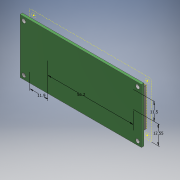
# Autodesk Inventor part: LCD Display
Saved by Autodesk Inventor 2017 (Build 210142000, 142)
## iProperties
Created: 2017-07-31
Part Number: LCD Display
Material: Generic
Document SubType Name: Modeling
Designer: AlexS
Density: 1 g/cm^3
Appearance: Default
Author: AlexS
Autodesk Inventor part; units mm, degrees
ref_plane "YZ Plane" through (0, 0, 0) normal (1, 0, 0) x (0, 1, 0)
ref_plane "XZ Plane" through (0, 0, 0) normal (0, 1, 0) x (-1, 0, 0)
ref_plane "XY Plane" through (0, 0, 0) normal (0, 0, 1) x (1, 0, 0)
sketch "Sketch1" plane through (0, 0, 0) normal (0, 1, 0) x (-1, 0, 0)
  line L0 (-40, 18) -> (40, 18)
  line L1 (40, 18) -> (40, -18)
  line L2 (40, -18) -> (-40, -18)
  line L3 (-40, -18) -> (-40, 18)
  line L4 (-40, 18) -> (40, -18) construction
  line L5 (40, 18) -> (-40, -18) construction
  point P0 (0, 0)
  dimension "d0" = 80
  dimension "d1" = 36
  constraints: 12 end point, 2 midpoint, 2 parallel, 1 horizontal, 1 perpendicular
  measures "d0" distance of L1.end L2.end
  measures "d1" distance of L0.end L1.end
extrude "Extrusion1" add sketch "Sketch1" along normal blind 1.6
sketch "Sketch2" plane through (0, 1.6, 0) normal (0, 1, 0) x (1, 0, 0)
  line L0 (-40, -18) -> (40, -18) construction
  line L1 (40, -18) -> (40, 18) construction
  line L2 (40, 18) -> (-40, 18) construction
  line L3 (-40, 18) -> (-40, -18) construction
  point P0 (0, 0)
  point P1 (-37.5, 15.5)
  point P2 (37.5, 15.5)
  point P3 (-37.5, -15.5)
  point P4 (37.5, -15.5)
  dimension "d4" = 75
  dimension "d5" = 31
  dimension "d6" = 2.5
  dimension "d7" = 2.5
  constraints: 2 horizontal alignment, 2 vertical alignment
  measures "d4" distance of point (37.5, 15.5) point (-37.5, 15.5)
  measures "d5" distance of point (-37.5, 15.5) point (-37.5, -15.5)
  measures "d6" distance from line of L3 point (-37.5, 15.5)
  measures "d7" distance from line of L2 point (-37.5, 15.5)
hole "Hole1" at (-37.5, 1.6, -15.5) at (37.5, 1.6, -15.5) at (-37.5, 1.6, 15.5) at (37.5, 1.6, 15.5) direction (0, -1, 0) diameter 2.5 end through all
sketch "Sketch3" plane through (0, 1.6, 0) normal (0, 1, 0) x (1, 0, 0)
  line L0 (36.85, -12.7) -> (-36.85, -12.7)
  line L1 (-36.85, -12.7) -> (-36.85, 12.1)
  line L2 (-36.85, 12.1) -> (36.85, 12.1)
  line L3 (36.85, 12.1) -> (36.85, -12.7)
  line L4 (36.85, -12.7) -> (-36.85, 12.1) construction
  line L5 (-36.85, -12.7) -> (36.85, 12.1) construction
  circle A0 centre (-37.5, -15.5) radius 1.25 construction
  circle A1 centre (-37.5, 15.5) radius 1.25 construction
  circle A2 centre (37.5, 15.5) radius 1.25 construction
  circle A3 centre (37.5, -15.5) radius 1.25 construction
  line L6 (-40, -18) -> (40, -18) construction
  line L7 (40, -18) -> (40, 18) construction
  line L8 (40, 18) -> (-40, 18) construction
  line L9 (-40, 18) -> (-40, -18) construction
  point P0 (0, 0)
  point P1 (0, -0.3)
  dimension "d15" = 73.7
  dimension "d16" = 24.8
  dimension "d17" = 5.9
  dimension "d18" = 3.15
  constraints: 12 end point, 2 midpoint, 2 parallel, 1 horizontal, 1 perpendicular
  measures "d15" distance of L1.end L2.end
  measures "d16" distance of L0.end L1.end
  measures "d17" distance between parallel lines of L8 L2
  measures "d18" distance between parallel lines of L9 L1
extrude "Extrusion2" add sketch "Sketch3" along normal blind 5
sketch "Sketch4" plane through (0, 6.6, 0) normal (0, 1, 0) x (1, 0, 0)
  line L0 (32.25, -7.7) -> (-32.25, -7.7)
  line L1 (-32.25, -7.7) -> (-32.25, 7.1)
  line L2 (-32.25, 7.1) -> (32.25, 7.1)
  line L3 (32.25, 7.1) -> (32.25, -7.7)
  line L4 (32.25, -7.7) -> (-32.25, 7.1) construction
  line L5 (-32.25, -7.7) -> (32.25, 7.1) construction
  line L6 (-36.85, -12.7) -> (-36.85, 12.1) construction
  line L7 (-36.85, 12.1) -> (36.85, 12.1) construction
  line L8 (36.85, 12.1) -> (36.85, -12.7) construction
  line L9 (36.85, -12.7) -> (-36.85, -12.7) construction
  circle A0 centre (-37.5, -15.5) radius 1.25 construction
  circle A1 centre (-37.5, 15.5) radius 1.25 construction
  circle A2 centre (37.5, 15.5) radius 1.25 construction
  circle A3 centre (37.5, -15.5) radius 1.25 construction
  line L10 (-40, -18) -> (40, -18) construction
  line L11 (40, -18) -> (40, 18) construction
  line L12 (40, 18) -> (-40, 18) construction
  line L13 (-40, 18) -> (-40, -18) construction
  point P0 (0, 0)
  point P1 (0, -0.3)
  dimension "d21" = 64.5
  dimension "d22" = 14.8
  dimension "d23" = 10.9
  dimension "d24" = 7.75
  constraints: 12 end point, 2 midpoint, 2 parallel, 1 horizontal, 1 perpendicular
  measures "d21" distance of L0.start L0.end
  measures "d22" distance of L0.end L1.end
  measures "d23" distance between parallel lines of L12 L2
  measures "d24" distance between parallel lines of L13 L1
extrude "Extrusion3" cut sketch "Sketch4" against normal blind 0.1
sketch "Sketch5" plane through (0, 6.5, 0) normal (0, 1, 0) x (1, 0, 0)
  line L0 (-28.1, 5.45) -> (28.1, 5.45) construction
  line L1 (28.1, 5.45) -> (28.1, -6.05) construction
  line L2 (28.1, -6.05) -> (-28.1, -6.05) construction
  line L3 (-28.1, -6.05) -> (-28.1, 5.45) construction
  line L4 (32.25, -7.7) -> (-32.25, -7.7) construction
  line L5 (32.25, 7.1) -> (32.25, -7.7) construction
  line L6 (-32.25, 7.1) -> (32.25, 7.1) construction
  line L7 (-32.25, -7.7) -> (-32.25, 7.1) construction
  line L8 (-36.85, -12.7) -> (-36.85, 12.1) construction
  line L9 (-36.85, 12.1) -> (36.85, 12.1) construction
  line L10 (36.85, 12.1) -> (36.85, -12.7) construction
  line L11 (36.85, -12.7) -> (-36.85, -12.7) construction
  circle A0 centre (-37.5, -15.5) radius 1.25 construction
  circle A1 centre (-37.5, 15.5) radius 1.25 construction
  circle A2 centre (37.5, 15.5) radius 1.25 construction
  circle A3 centre (37.5, -15.5) radius 1.25 construction
  line L12 (-40, -18) -> (40, -18) construction
  line L13 (40, -18) -> (40, 18) construction
  line L14 (40, 18) -> (-40, 18) construction
  line L15 (-40, 18) -> (-40, -18) construction
  line L16 (32.25, 7.1) -> (32.25, -7.7) construction
  line L17 (32.25, -7.7) -> (-32.25, -7.7) construction
  line L18 (-32.25, -7.7) -> (-32.25, 7.1) construction
  line L19 (-32.25, 7.1) -> (32.25, 7.1) construction
  line L20 (-36.85, -12.7) -> (36.85, -12.7) construction
  line L21 (36.85, -12.7) -> (36.85, 12.1) construction
  line L22 (36.85, 12.1) -> (-36.85, 12.1) construction
  line L23 (-36.85, 12.1) -> (-36.85, -12.7) construction
  point P0 (0, 0)
  dimension "d27" = 56.2
  dimension "d28" = 11.5
  dimension "d29" = 12.55
  dimension "d30" = 11.9
  constraints: 2 other
  measures "d27" distance of L0.start L0.end
  measures "d28" distance of L0.end L1.end
  measures "d29" distance between parallel lines of L14 L0
  measures "d30" distance between parallel lines of L15 L3
body "Solid1"
